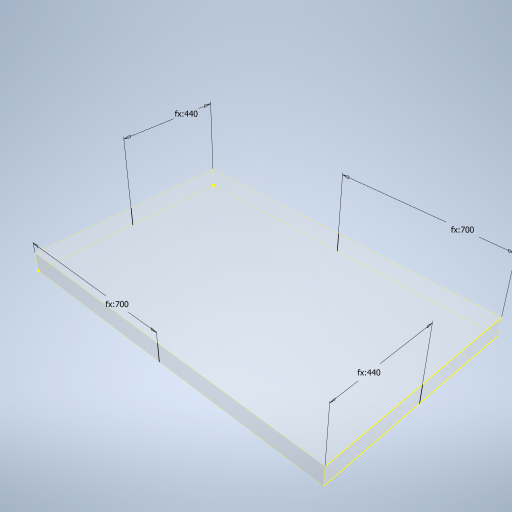
# Autodesk Inventor part: Rahmen
Saved by Autodesk Inventor 2024 (Build 280153020, 153B)
## iProperties
Created: 2023-08-07
Part Number: Rahmen
Material: Generisch
Document SubType Name: Modeling
Designer: hol
Density: 1 g/cm^3
Appearance: Polycarbonat - klar
FrameZdist: 80,000 mm
FrameXdist: 880,000 mm
FrameYdist: 1400,000 mm
Author: hol
Autodesk Inventor part; units mm, degrees
ref_plane "YZ Plane" through (0, 0, 0) normal (1, 0, 0) x (0, 1, 0)
ref_plane "XZ Plane" through (0, 0, 0) normal (0, 1, 0) x (-1, 0, 0)
ref_plane "XY Plane" through (0, 0, 0) normal (0, 0, 1) x (1, 0, 0)
sketch "Skizze1" plane through (0, 0, 0) normal (0, 1, 0) x (-1, 0, 0)
  line L0 (0, 0) -> (-1400, 0)
  line L1 (-1400, 0) -> (-1400, -880)
  line L2 (-1400, -880) -> (0, -880)
  line L3 (0, -880) -> (0, 0)
  dimension "Y" = 1400
  dimension "X" = 880
  constraints: 8 end point, 2 parallel, 1 horizontal, 1 perpendicular
  measures "Y" distance of L2.end L1.end
  measures "X" distance of L1.end L0.end
extrude "Extrusion1" add sketch "Skizze1" along normal blind 80
sketch "Skizze6" plane through (0, 0, 0) normal (0, 0, 1) x (1, 0, 0)
  line L0 (0, 0) -> (1400, 0) construction
  line L1 (1400, 0) -> (1400, 80) construction
  line L2 (0, 80) -> (1400, 80) construction
  line L3 (0, 0) -> (0, 80) construction
  line L4 (700, 80) -> (700, 0)
  dimension "d44" = 700
  constraints: 2 end point, 2 midpoint, 1 perpendicular
  measures "d44" distance from line of L4 L2.start
sketch "Skizze7" plane through (1400, 0, 0) normal (1, 0, 0) x (0, 0, -1)
  line L0 (0, 0) -> (880, 0) construction
  line L1 (880, 0) -> (880, 80) construction
  line L2 (0, 80) -> (880, 80) construction
  line L3 (0, 0) -> (0, 80) construction
  line L4 (880, 80) -> (0, 80) projected
  line L5 (440, 80) -> (440, 0)
  line L6 (0, 0) -> (880, 0) projected
  dimension "d45" = 440
  constraints: 2 end point, 2 midpoint, 1 vertical
  measures "d45" distance from line of L3 L5.start
sketch "Skizze8" plane through (1400, 0, -880) normal (0, 0, -1) x (-1, 0, 0)
  line L0 (0, 0) -> (1400, 0) construction
  line L1 (1400, 0) -> (1400, 80) construction
  line L2 (0, 80) -> (1400, 80) construction
  line L3 (0, 0) -> (0, 80) construction
  line L4 (700, 80) -> (700, 0)
  dimension "d46" = 700
  constraints: 2 end point, 2 midpoint, 1 perpendicular
  measures "d46" distance from line of L3 L4.start
sketch "Skizze9" plane through (0, 0, -880) normal (-1, 0, 0) x (0, 0, 1)
  line L0 (0, 0) -> (880, 0) construction
  line L1 (880, 0) -> (880, 80) construction
  line L2 (0, 80) -> (880, 80) construction
  line L3 (0, 0) -> (0, 80) construction
  line L4 (440, 80) -> (440, 0)
  dimension "d47" = 440
  constraints: 2 end point, 2 midpoint, 1 perpendicular
  measures "d47" distance of L2.start L4.start
equation "\"Y\" = FrameYdist"
equation "\"X\" = FrameXdist"
equation "\"Z\" = FrameZdist"
equation "\"d44\" = 0.5 * Y"
equation "\"d45\" = 0.5 * X"
equation "\"d46\" = 0.5 * Y"
equation "\"d47\" = 0.5 * X"
equation "\"FrameZdist\" = FrameZdist_1"
equation "\"FrameXdist\" = FrameXdist_1"
equation "\"FrameYdist\" = FrameYdist_1"
equation "\"FrameZdist_1\" = 80"
equation "\"FrameXdist_1\" = 880"
equation "\"FrameYdist_1\" = 1400"
